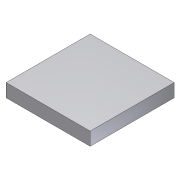
# Autodesk Inventor part: RX_tan_U7_MBC13917
Saved by Autodesk Inventor 2014 SP1 (Build 180222100, 222)
## iProperties
Created: 2013-10-12
Part Number: RX_tan_U7_MBC13917
Document SubType Name: Modeling
Designer: Robert Davis
Density: 1 g/cm^3
Material: Generic
Appearance: Default
Author: Robert Davis
Autodesk Inventor part; units mm, degrees
ref_plane "YZ Plane" through (0, 0, 0) normal (1, 0, 0) x (0, 1, 0)
ref_plane "XZ Plane" through (0, 0, 0) normal (0, 1, 0) x (-1, 0, 0)
ref_plane "XY Plane" through (0, 0, 0) normal (0, 0, 1) x (1, 0, 0)
sketch "Sketch1" plane through (0, 0, 0) normal (0, 0, 1) x (1, 0, 0)
  line L0 (3.175, -3.175) -> (3.175, 3.175)
  line L1 (3.175, 3.175) -> (-3.175, 3.175)
  line L2 (-3.175, 3.175) -> (-3.175, -3.175)
  line L3 (-3.175, -3.175) -> (3.175, -3.175)
  line L4 (0, 0) -> (1.3238, 0)
  line L5 (0, 0) -> (0, 0.8095)
  dimension "d0" = 6.35
  dimension "d1" = 6.35
  constraints: 12 end point, 3 horizontal, 3 vertical, 1 coincident, 2 other
  measures "d0" distance of L1.end L2.end
  measures "d1" distance of L0.end L1.end
extrude "Extrusion1" add sketch "Sketch1" along normal blind 1
body "Solid1"
